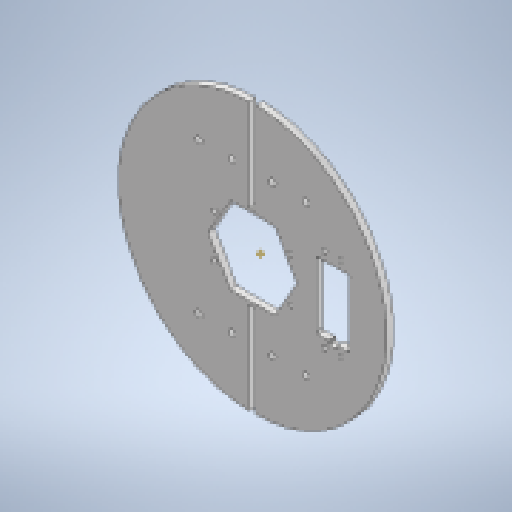
# Autodesk Inventor part: лицо1
Saved by Autodesk Inventor 2023.1 (Build 271208000, 208)
## iProperties
Created: 2024-12-06
Part Number: лицо1
Material: Типовые
Document SubType Name: Modeling
Designer: DELL
Density: 1 g/cm^3
Appearance: По умолчанию
Author: DELL
Autodesk Inventor part; units mm, degrees
ref_plane "YZ Plane" through (0, 0, 0) normal (1, 0, 0) x (0, 1, 0)
ref_plane "XZ Plane" through (0, 0, 0) normal (0, 1, 0) x (-1, 0, 0)
ref_plane "XY Plane" through (0, 0, 0) normal (0, 0, 1) x (1, 0, 0)
sketch "Эскиз1" plane through (0, 0, 0) normal (0, 0, 1) x (1, 0, 0)
  circle A0 centre (0, 0) radius 80
  line L0 (26.5581, 0) -> (13.2791, -23)
  line L1 (13.2791, -23) -> (-13.2791, -23)
  line L2 (-13.2791, -23) -> (-26.5581, 0)
  line L3 (-26.5581, 0) -> (-13.2791, 23)
  line L4 (-13.2791, 23) -> (13.2791, 23)
  line L5 (13.2791, 23) -> (26.5581, 0)
  dimension "d49" = 160
  dimension "d50" = 46
  constraints: 12 end point, 2 coincident, 1 centre point, 13 other
  measures "d49" diameter of A0
  measures "d50" distance between parallel lines of L4 L1
extrude "Выдавливание1" add sketch "Эскиз1" along normal blind 4
sketch "Эскиз2" plane through (0, 0, 0) normal (0, 0, -1) x (-1, 0, 0)
  circle A0 centre (0, 0) radius 80 projected
  line L0 (0, 80) -> (0, -80) construction
  line L1 (2, -80) -> (-2, -80)
  line L2 (-2, -80) -> (-2, 80)
  line L3 (-2, 80) -> (2, 80)
  line L4 (2, 80) -> (2, -80)
  line L5 (2, -80) -> (-2, 80) construction
  line L6 (-2, -80) -> (2, 80) construction
  line L7 (-2, 25) -> (2, 25)
  line L8 (-2, -25) -> (2, -25)
  point P0 (0, -25)
  point P1 (0, 80)
  point P2 (0, 25)
  dimension "d2" = 4
  dimension "d3" = 160
  dimension "d4" = 55
  dimension "d5" = 55
  constraints: 18 end point, 5 midpoint, 4 point on line, 3 perpendicular, 2 parallel, 2 point on circle, 1 horizontal, 1 vertical
  measures "d2" distance of L2.end L3.end
  measures "d3" distance of L1.end L2.end
  measures "d4" distance from line of L1 point (0, -25)
  measures "d5" distance of point (0, 80) point (0, 25)
extrude "Выдавливание2" cut sketch "Эскиз2" against normal blind 10 contours L4 L7 L2 A0 | A0 L3 L4 | L4 L1 A0 | A0 L2 L8 L4 | A0 L2 L3 | L1 L2 A0
sketch "Эскиз4" plane through (0, 0, 4) normal (0, 0, 1) x (1, 0, 0)
  line L0 (57, 20) -> (39, 20)
  line L1 (38, 19) -> (38, -19)
  line L2 (58, -19) -> (58, 19)
  arc A0 (39, 20) -> (38, 19) centre (39, 19) ccw
  arc A1 (38, -19) -> (39, -20) centre (39, -19) ccw
  arc A2 (57, -20) -> (58, -19) centre (57, -19) ccw
  arc A3 (58, 19) -> (57, 20) centre (57, 19) ccw
  line L3 (45.7, -22) -> (50.3, -22)
  line L4 (50.5, -21.8) -> (50.5, -20.2)
  line L5 (50.5, -20) -> (48, -20) construction
  line L6 (45.5, -20.2) -> (45.5, -21.8)
  line L7 (50.5, -20) -> (45.5, -22) construction
  line L8 (48, -21) -> (48, -20) construction
  line L9 (0, 0) -> (112.2307, 0) construction
  line L10 (57.7071, 19.7071) -> (38.2929, -19.7071) construction
  line L11 (38.2929, 19.7071) -> (57.7071, -19.7071) construction
  line L12 (48, 20) -> (48, -20) construction
  line L13 (39, -20) -> (45.3, -20)
  line L14 (50.7, -20) -> (57, -20)
  arc A4 (50.7, -20) -> (50.5, -20.2) centre (50.7, -20.2) ccw
  arc A5 (45.5, -20.2) -> (45.3, -20) centre (45.3, -20.2) ccw
  arc A6 (45.5, -21.8) -> (45.7, -22) centre (45.7, -21.8) ccw
  arc A7 (50.3, -22) -> (50.5, -21.8) centre (50.3, -21.8) ccw
  line L15 (0, 0) -> (0, 111.2909) construction
  line L16 (48, -20) -> (48, -24.7856) construction
  point P0 (47.3361, 0)
  point P1 (50.5, -22)
  point P2 (45.5, -20)
  point P3 (48, 0)
  dimension "d35" = 1
  dimension "d40" = 5
  dimension "d41" = 2
  dimension "d42" = 20
  dimension "d44" = 38
  dimension "d45" = 0.2
  dimension "d46" = 38
  constraints: 34 end point, 20 point on circle, 18 tangent, 11 point on line, 8 centre point, 7 parallel, 6 equal radius, 3 coincident, 3 horizontal, 3 midpoint, 2 perpendicular, 2 vertical
  measures "d35" radius of A0
  measures "d40" distance of L5.start point (45.5, -20)
  measures "d41" distance of L5.start point (50.5, -22)
  measures "d42" distance between parallel lines of L2 L1
  measures "d44" distance from line of L1 L9.start
  measures "d45" radius of A4
  measures "d46" distance of L2.start L2.end
extrude "Выдавливание4" cut sketch "Эскиз4" against normal blind 10
sketch "Эскиз6" plane through (0, 0, 4) normal (0, 0, 1) x (1, 0, 0)
  circle A0 centre (43, -25) radius 1.5
  circle A1 centre (53, -25) radius 1.5
  line L0 (43, -25) -> (53, -25) construction
  line L1 (53, -25) -> (53, 25) construction
  line L2 (53, 25) -> (43, 25) construction
  line L3 (43, 25) -> (43, -25) construction
  line L4 (43, -25) -> (53, 25) construction
  circle A2 centre (43, 25) radius 1.5
  circle A3 centre (53, 25) radius 1.5
  arc A4 (39, 20) -> (38, 19) centre (39, 19) ccw projected
  arc A5 (57, -20) -> (58, -19) centre (57, -19) ccw projected
  line L5 (39, 19) -> (57, -19) construction
  point P0 (0, 0)
  point P1 (48, 0)
  dimension "d15" = 3
  dimension "d16" = 50
  dimension "d17" = 10
  dimension "d20" = 3
  dimension "d21" = 3
  dimension "d22" = 3
  constraints: 12 end point, 4 centre point, 3 perpendicular, 2 coincident, 2 midpoint, 1 horizontal
  measures "d15" diameter of A0
  measures "d16" distance of L0.end L1.end
  measures "d17" distance of L1.end L2.end
  measures "d20" diameter of A2
  measures "d21" diameter of A3
  measures "d22" diameter of A1
extrude "Выдавливание5" cut sketch "Эскиз6" against normal blind 10
sketch "Эскиз8" plane through (0, 0, 4) normal (0, 0, 1) x (1, 0, 0)
  circle A0 centre (-32, 44.908) radius 2.55 construction
  circle A1 centre (-12, 44.908) radius 2.55 construction
  circle A2 centre (12, 44.908) radius 2.55 construction
  circle A3 centre (32, 44.908) radius 2.55 construction
  circle A4 centre (32, -44.908) radius 2.55 construction
  circle A5 centre (12, -44.908) radius 2.55 construction
  circle A6 centre (-32, -44.908) radius 2.55 construction
  circle A7 centre (-12, -44.908) radius 2.55 construction
  circle A8 centre (-32, 44.908) radius 1.95
  circle A9 centre (-12, 44.908) radius 1.95
  circle A10 centre (12, 44.908) radius 1.95
  circle A11 centre (32, 44.908) radius 1.95
  circle A12 centre (-32, -44.908) radius 1.95
  circle A13 centre (-12, -44.908) radius 1.95
  circle A14 centre (12, -44.908) radius 1.95
  circle A15 centre (32, -44.908) radius 1.95
  point P0 (0, 0)
  dimension "d23" = 3.9
  dimension "d24" = 3.9
  dimension "d25" = 3.9
  dimension "d26" = 3.9
  dimension "d27" = 3.9
  dimension "d28" = 3.9
  dimension "d29" = 3.9
  dimension "d30" = 3.9
  constraints: 8 centre point, 8 coincident
  measures "d23" diameter of A8
  measures "d24" diameter of A9
  measures "d25" diameter of A10
  measures "d26" diameter of A11
  measures "d27" diameter of A12
  measures "d28" diameter of A13
  measures "d29" diameter of A14
  measures "d30" diameter of A15
extrude "Выдавливание6" cut sketch "Эскиз8" against normal blind 10
sketch "Эскиз9" plane through (0, 0, 0) normal (0, 0, -1) x (-1, 0, 0)
  circle A0 centre (-22.5167, -13) radius 1.5
  circle A1 centre (-22.5167, 13) radius 1.5
  circle A2 centre (0, 0) radius 26 construction
  circle A3 centre (22.5167, 13) radius 1.5
  circle A4 centre (-22.5167, 13) radius 1.5
  circle A5 centre (22.5167, 13) radius 1.5
  circle A6 centre (22.5167, -13) radius 1.5
  point P0 (0, 0)
extrude "Выдавливание7" cut sketch "Эскиз9" against normal blind 10
